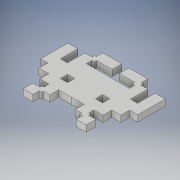
# Autodesk Inventor part: Monster2
Saved by Autodesk Inventor 2019 (Build 230136000, 136)
## iProperties
Created: 2018-12-03
Part Number: Monster2
Material: Generic
Document SubType Name: Modeling
Designer: Administrator
Density: 1 g/cm^3
Appearance: Default
Author: Administrator
Autodesk Inventor part; units mm, degrees
ref_plane "YZ Plane" through (0, 0, 0) normal (1, 0, 0) x (0, 1, 0)
ref_plane "XZ Plane" through (0, 0, 0) normal (0, 1, 0) x (-1, 0, 0)
ref_plane "XY Plane" through (0, 0, 0) normal (0, 0, 1) x (1, 0, 0)
sketch "Sketch1" plane through (0, 0, 0) normal (0, 1, 0) x (-1, 0, 0)
  line L0 (0, 0) -> (464.159, 0) construction
  line L1 (464.159, 0) -> (464.159, -207.7664) construction
  line L2 (464.159, -207.7664) -> (0, -207.7664) construction
  line L3 (0, -207.7664) -> (0, 0) construction
  line L4 (89.199, -168.5726) -> (89.199, -173.9719)
  line L5 (89.199, -173.9719) -> (86.6636, -173.9719)
  line L6 (86.6636, -173.9719) -> (86.6636, -176.4581)
  line L7 (86.6636, -176.4581) -> (71.2328, -176.4581)
  line L8 (71.2328, -176.4581) -> (71.2328, -186.2934)
  line L9 (71.2328, -186.2934) -> (90.3359, -186.2934)
  line L10 (90.3359, -186.2934) -> (90.3359, -179.7626)
  line L11 (90.3359, -179.7626) -> (92.1613, -179.7626)
  line L12 (92.1613, -179.7626) -> (92.1613, -177.2606)
  line L13 (92.1613, -177.2606) -> (99.2738, -177.2606)
  line L14 (99.2738, -177.2606) -> (99.2738, -159.6681)
  line L15 (99.2738, -159.6681) -> (106.4808, -159.6681)
  line L16 (106.4808, -159.6681) -> (106.4808, -177.355)
  line L17 (106.4808, -177.355) -> (116.4572, -177.355)
  line L18 (116.4572, -177.355) -> (116.4572, -149.6917)
  line L19 (116.4572, -149.6917) -> (109.1915, -149.6917)
  line L20 (109.1915, -149.6917) -> (109.1915, -140.7968)
  line L21 (109.1915, -140.7968) -> (99.2738, -140.7968)
  line L22 (99.2738, -140.7968) -> (99.2738, -131.8637)
  line L23 (99.2738, -131.8637) -> (90.1524, -131.8637)
  line L24 (90.1524, -131.8637) -> (90.1524, -126.827)
  line L25 (90.1524, -126.827) -> (92.1613, -126.827)
  line L26 (92.1613, -126.827) -> (92.1613, -124.6793)
  line L27 (92.1613, -124.6793) -> (99.2738, -124.6793)
  line L28 (99.2738, -124.6793) -> (99.2738, -114.8781)
  line L29 (99.2738, -114.8781) -> (89.326, -114.8781)
  line L30 (89.326, -114.8781) -> (89.326, -121.2519)
  line L31 (89.326, -121.2519) -> (86.6636, -121.2519)
  line L32 (86.6636, -121.2519) -> (86.6636, -122.9811)
  line L33 (86.6636, -122.9811) -> (80.2684, -122.9811)
  line L34 (80.2684, -122.9811) -> (80.2684, -131.8637)
  line L35 (67.5567, -131.8637) -> (80.2684, -131.8637)
  line L36 (67.602, -168.5726) -> (89.199, -168.5726)
  line L37 (46.005, -168.6259) -> (46.0183, -174.0251)
  line L38 (46.0183, -174.0251) -> (48.5537, -174.0188)
  line L39 (48.5537, -174.0188) -> (48.5598, -176.5051)
  line L40 (48.5598, -176.5051) -> (63.9906, -176.467)
  line L41 (63.9906, -176.467) -> (64.0148, -186.3023)
  line L42 (64.0148, -186.3023) -> (44.9117, -186.3494)
  line L43 (44.9117, -186.3494) -> (44.8956, -179.8186)
  line L44 (44.8956, -179.8186) -> (43.0703, -179.8231)
  line L45 (43.0703, -179.8231) -> (43.0641, -177.3211)
  line L46 (43.0641, -177.3211) -> (35.9516, -177.3387)
  line L47 (35.9516, -177.3387) -> (35.9083, -159.7462)
  line L48 (35.9083, -159.7462) -> (28.7013, -159.7639)
  line L49 (28.7013, -159.7639) -> (28.7449, -177.4508)
  line L50 (28.7449, -177.4508) -> (18.7685, -177.4754)
  line L51 (18.7685, -177.4754) -> (18.7003, -149.8121)
  line L52 (18.7003, -149.8121) -> (26.8729, -149.792)
  line L53 (26.8729, -149.792) -> (26.8509, -140.8972)
  line L54 (26.8509, -140.8972) -> (35.8617, -140.875)
  line L55 (35.8617, -140.875) -> (35.8397, -131.9419)
  line L56 (35.8397, -131.9419) -> (44.9611, -131.9194)
  line L57 (44.9611, -131.9194) -> (44.9487, -126.8827)
  line L58 (44.9487, -126.8827) -> (42.9398, -126.8877)
  line L59 (42.9398, -126.8877) -> (42.9345, -124.7399)
  line L60 (42.9345, -124.7399) -> (35.822, -124.7574)
  line L61 (35.822, -124.7574) -> (35.7979, -114.9563)
  line L62 (35.7979, -114.9563) -> (45.7457, -114.9318)
  line L63 (45.7457, -114.9318) -> (45.7614, -121.3056)
  line L64 (45.7614, -121.3056) -> (48.4237, -121.299)
  line L65 (48.4237, -121.299) -> (48.428, -123.0282)
  line L66 (48.428, -123.0282) -> (54.8232, -123.0124)
  line L67 (54.8232, -123.0124) -> (54.8451, -131.8951)
  line L68 (67.5567, -131.8637) -> (54.8451, -131.8951)
  line L69 (67.602, -168.5726) -> (46.005, -168.6259)
  line L70 (46.7205, -142.4875) -> (53.9587, -142.4875)
  line L71 (53.9587, -142.4875) -> (53.9587, -149.7258)
  line L72 (53.9587, -149.7258) -> (46.7205, -149.7258)
  line L73 (46.7205, -149.7258) -> (46.7205, -142.4875)
  line L74 (82.0966, -142.4875) -> (89.3348, -142.4875)
  line L75 (89.3348, -142.4875) -> (89.3348, -149.7258)
  line L76 (89.3348, -149.7258) -> (82.0966, -149.7258)
  line L77 (82.0966, -149.7258) -> (82.0966, -142.4875)
  dimension "d30" = 90
  dimension "d32" = 90
  dimension "d34" = 90
  dimension "d35" = 90
  dimension "d36" = 7.2382
  dimension "d39" = 7.2382
  dimension "d40" = 7.2382
  dimension "d41" = 7.2382
  dimension "d43" = 19.8567
  dimension "d44" = 28.1378
  constraints: 148 end point, 26 perpendicular, 8 horizontal, 8 point on line, 4 parallel, 2 other
  measures "d30" angle of L7 L8
  measures "d32" angle of L57 L56
  measures "d34" angle of L55 L54
  measures "d35" angle of L56 L55
  measures "d36" distance of L72.end L70.start
  measures "d39" distance of L71.end L72.end
  measures "d40" distance of L75.end L76.end
  measures "d41" distance of L76.end L74.start
  measures "d43" distance between parallel lines of L20 L75
  measures "d44" distance between parallel lines of L71 L77
extrude "Extrusion1" add sketch "Sketch1" along normal blind 6.35
equation "\"d39\" = d36"
equation "\"d40\" = d36"
body "Solid1"
